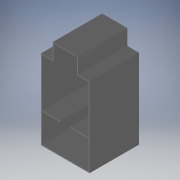
# Autodesk Inventor part: Main
Saved by Autodesk Inventor 2020 (Build 240168000, 168)
## iProperties
Created: 2019-09-17
Part Number: Main
Material: 일반
Document SubType Name: Modeling
Designer: Knowblesse
Density: 1 g/cm^3
Appearance: 기본값
Author: Knowblesse
Autodesk Inventor part; units mm, degrees
ref_plane "YZ Plane" through (0, 0, 0) normal (1, 0, 0) x (0, 1, 0)
ref_plane "XZ Plane" through (0, 0, 0) normal (0, 1, 0) x (-1, 0, 0)
ref_plane "XY Plane" through (0, 0, 0) normal (0, 0, 1) x (1, 0, 0)
sketch "스케치1" plane through (0, 0, 0) normal (0, 0, 1) x (1, 0, 0)
  line L0 (0, 0) -> (500, 0)
  line L1 (500, 0) -> (500, 820)
  line L2 (0, 0) -> (0, 820)
  line L3 (0, 820) -> (120, 820)
  line L4 (120, 820) -> (120, 980)
  line L5 (120, 980) -> (380, 980)
  line L6 (380, 980) -> (380, 820)
  line L7 (380, 820) -> (500, 820)
  line L8 (10, 10) -> (490, 10)
  line L9 (490, 10) -> (490, 305)
  line L10 (490, 305) -> (300, 305)
  line L11 (300, 305) -> (300, 315)
  line L12 (300, 315) -> (490, 315)
  line L13 (490, 315) -> (490, 810)
  line L14 (490, 810) -> (370, 810)
  line L15 (370, 810) -> (370, 970)
  line L16 (370, 970) -> (130, 970)
  line L17 (130, 970) -> (130, 810)
  line L18 (130, 810) -> (10, 810)
  line L19 (10, 810) -> (10, 315)
  line L20 (10, 315) -> (200, 315)
  line L21 (200, 315) -> (200, 305)
  line L22 (200, 305) -> (10, 305)
  line L23 (10, 305) -> (10, 10)
  dimension "d0" = 500
  dimension "d1" = 820
  dimension "d2" = 820
  dimension "d3" = 10
  dimension "d4" = 10
  dimension "d5" = 10
  dimension "d6" = 10
  dimension "d7" = 10
  dimension "d8" = 10
  dimension "d9" = 10
  dimension "d10" = 10
  dimension "d11" = 100
  dimension "d12" = 295
  dimension "d13" = 240
  dimension "d14" = 160
  constraints: 48 end point, 15 perpendicular, 10 point on line, 2 collinear, 2 horizontal, 1 parallel, 1 vertical
  measures "d0" distance of L0.start L0.end
  measures "d1" distance of L0.end L1.end
  measures "d2" distance of L0.start L2.end
  measures "d3" distance of L10.end L11.end
  measures "d4" distance between parallel lines of L2 L19
  measures "d5" distance between parallel lines of L1 L13
  measures "d6" distance between parallel lines of L5 L16
  measures "d7" distance between parallel lines of L3 L18
  measures "d8" distance between parallel lines of L6 L15
  measures "d9" distance between parallel lines of L4 L17
  measures "d10" distance between parallel lines of L0 L8
  measures "d11" distance between parallel lines of L11 L21
  measures "d12" distance between parallel lines of L8 L10
  measures "d13" distance between parallel lines of L15 L17
  measures "d14" distance between parallel lines of L18 L16
extrude "돌출1" add sketch "스케치1" along normal blind 500
sketch "스케치2" plane through (0, 0, 0) normal (0, 0, -1) x (-1, 0, 0)
  line L0 (-380, 820) -> (-380, 980) projected
  line L1 (-500, 820) -> (-380, 820) projected
  line L2 (-500, 0) -> (-500, 820) projected
  line L3 (0, 0) -> (-500, 0) projected
  line L4 (0, 820) -> (0, 0) projected
  line L5 (-120, 820) -> (0, 820) projected
  line L6 (-120, 980) -> (-120, 820) projected
  line L7 (-380, 980) -> (-120, 980) projected
  line L8 (-490, 305) -> (-490, 10) projected
  line L9 (-300, 305) -> (-490, 305) projected
  line L10 (-300, 315) -> (-300, 305) projected
  line L11 (-490, 315) -> (-300, 315) projected
  line L12 (-490, 810) -> (-490, 315) projected
  line L13 (-370, 810) -> (-490, 810) projected
  line L14 (-370, 970) -> (-370, 810) projected
  line L15 (-130, 970) -> (-370, 970) projected
  line L16 (-130, 810) -> (-130, 970) projected
  line L17 (-10, 810) -> (-130, 810) projected
  line L18 (-10, 315) -> (-10, 810) projected
  line L19 (-200, 315) -> (-10, 315) projected
  line L20 (-200, 305) -> (-200, 315) projected
  line L21 (-10, 305) -> (-200, 305) projected
  line L22 (-10, 10) -> (-10, 305) projected
  line L23 (-490, 10) -> (-10, 10) projected
extrude "돌출2" add sketch "스케치2" along normal blind 10 contours L0 L7 L6 L5 L4 L3 L2 L1 | L9 L10 L11 L12 L13 L14 L15 L16 L17 L18 L19 L20 L21 L22 L23 L8
sketch "스케치3" plane through (0, 0, 500) normal (0, 0, 1) x (1, 0, 0)
  line L0 (380, 820) -> (380, 980) projected
  line L1 (380, 980) -> (120, 980) projected
  line L2 (120, 980) -> (120, 820) projected
  line L3 (120, 820) -> (0, 820) projected
  line L4 (0, 820) -> (0, 0) projected
  line L5 (0, 0) -> (500, 0) projected
  line L6 (500, 0) -> (500, 820) projected
  line L7 (500, 820) -> (380, 820) projected
  line L8 (490, 305) -> (490, 10) projected
  line L9 (490, 10) -> (10, 10) projected
  line L10 (10, 10) -> (10, 305) projected
  line L11 (10, 305) -> (200, 305) projected
  line L12 (200, 305) -> (200, 315) projected
  line L13 (200, 315) -> (10, 315) projected
  line L14 (10, 315) -> (10, 810) projected
  line L15 (10, 810) -> (130, 810) projected
  line L16 (130, 810) -> (130, 970) projected
  line L17 (130, 970) -> (370, 970) projected
  line L18 (370, 970) -> (370, 810) projected
  line L19 (370, 810) -> (490, 810) projected
  line L20 (490, 810) -> (490, 315) projected
  line L21 (490, 315) -> (300, 315) projected
  line L22 (300, 315) -> (300, 305) projected
  line L23 (300, 305) -> (490, 305) projected
  line L24 (120, 980) -> (120, 820) projected
  line L25 (380, 820) -> (380, 980) projected
  line L26 (120, 960) -> (380, 960)
  line L27 (380, 960) -> (380, 970)
  line L28 (380, 970) -> (120, 970)
  line L29 (120, 970) -> (120, 960)
  line L30 (130, 970) -> (370, 970) projected
  point P0 (370, 960)
  point P1 (130, 960)
  dimension "d19" = 10
  constraints: 8 end point, 2 parallel, 2 point on line, 1 collinear, 1 horizontal, 1 perpendicular
  measures "d19" distance of L27.end L26.end
extrude "돌출3" cut sketch "스케치3" against normal blind 250 contours L26 L18 L28 L0 | L26 L2 L28 L16
sketch "스케치4" plane through (380, 820, -10) normal (1, 0, 0) x (0, 0, -1)
  line L0 (0, 160) -> (0, 0) projected
  line L1 (0, 0) -> (-510, 0) projected
  line L2 (-40, 0) -> (-60, 0)
  line L3 (-60, 0) -> (-60, 10)
  line L4 (-60, 10) -> (-40, 10)
  line L5 (-40, 10) -> (-40, 0)
  line L6 (-10, -505) -> (-10, -10) projected
  point P0 (-10, -820)
  dimension "d22" = 20
  dimension "d23" = 10
  dimension "d24" = 30
  constraints: 8 end point, 2 parallel, 1 horizontal, 1 perpendicular, 1 point on line
  measures "d22" distance of L3.end L4.end
  measures "d23" distance of L2.end L3.end
  measures "d24" distance between parallel lines of L5 L6
extrude "돌출4" cut sketch "스케치4" against normal through all
sketch "스케치5" plane through (0, 0, 0) normal (0, 0, 1) x (1, 0, 0)
  point P0 (0, 0)
  point P1 (193.2447, 618.3101)
hole "구멍1" at (193.2447, 618.3101, 0) direction (0, 0, -1) diameter 1.5 end through all
